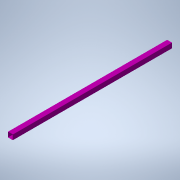
# Autodesk Inventor part: METALON_SUPORTE_CHAPA
Saved by Autodesk Inventor 2020 (Build 240168000, 168)
## iProperties
Created: 2016-02-21
Part Number: METALON_SUPORTE_CHAPA
Material: Genérico
Document SubType Name: Modeling
Designer: Everton
Density: 1 g/cm^3
Appearance: Padrão
Author: Everton
Autodesk Inventor part; units mm, degrees
ref_plane "YZ Plane" through (0, 0, 0) normal (1, 0, 0) x (0, 1, 0)
ref_plane "XZ Plane" through (0, 0, 0) normal (0, 1, 0) x (-1, 0, 0)
ref_plane "XY Plane" through (0, 0, 0) normal (0, 0, 1) x (1, 0, 0)
sketch "Sketch1" plane through (0, 0, 0) normal (0, 1, 0) x (-1, 0, 0)
  line L0 (20.1441, -11.0354) -> (20.1441, -47.0354)
  line L1 (18.1441, -49.0354) -> (-17.8559, -49.0354)
  line L2 (-19.8559, -47.0354) -> (-19.8559, -11.0354)
  line L3 (-17.8559, -9.0354) -> (18.1441, -9.0354)
  arc A0 (20.1441, -11.0354) -> (18.1441, -9.0354) centre (18.1441, -11.0354) ccw
  arc A1 (18.1441, -49.0354) -> (20.1441, -47.0354) centre (18.1441, -47.0354) ccw
  arc A2 (-17.8559, -9.0354) -> (-19.8559, -11.0354) centre (-17.8559, -11.0354) ccw
  arc A3 (-19.8559, -47.0354) -> (-17.8559, -49.0354) centre (-17.8559, -47.0354) ccw
  line L4 (18.6441, -47.0354) -> (18.6441, -11.0354)
  arc A4 (18.6441, -11.0354) -> (18.1441, -10.5354) centre (18.1441, -11.0354) ccw
  line L5 (18.1441, -10.5354) -> (-17.8559, -10.5354)
  arc A5 (-17.8559, -10.5354) -> (-18.3559, -11.0354) centre (-17.8559, -11.0354) ccw
  line L6 (-18.3559, -11.0354) -> (-18.3559, -47.0354)
  arc A6 (-18.3559, -47.0354) -> (-17.8559, -47.5354) centre (-17.8559, -47.0354) ccw
  line L7 (-17.8559, -47.5354) -> (18.1441, -47.5354)
  arc A7 (18.1441, -47.5354) -> (18.6441, -47.0354) centre (18.1441, -47.0354) ccw
  point P0 (0, 0)
  point P1 (20.1441, -9.0354)
  point P2 (20.1441, -49.0354)
  point P3 (-19.8559, -49.0354)
  dimension "d0" = 40
  dimension "d1" = 40
  dimension "d2" = 2
  dimension "d3" = 1.5
  constraints: 16 end point, 16 point on circle, 8 centre point, 8 tangent, 6 point on line, 4 perpendicular, 3 equal radius, 2 parallel, 1 vertical, 7 other
  measures "d0" distance of point (20.144, -9.035) point (20.144, -49.035)
  measures "d1" distance of point (20.144, -49.035) point (-19.856, -49.035)
  measures "d2" radius of A0
  measures "d3" distance between parallel lines of L0 L4
extrude "Extrusion1" add sketch "Sketch1" along normal blind 1260
body "Solid1"
